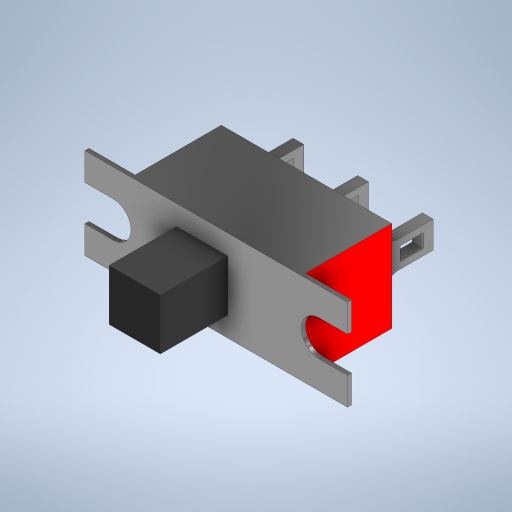
# Autodesk Inventor part: switch
Saved by Autodesk Inventor 2024 (Build 280153000, 153)
## iProperties
Created: 2023-11-08
Part Number: switch
Material: Všeobecné
Document SubType Name: Modeling
Designer: Simak
Density: 1 g/cm^3
Appearance: Výchozí
Author: Simak
Autodesk Inventor part; units mm, degrees
ref_plane "YZ Plane" through (0, 0, 0) normal (1, 0, 0) x (0, 1, 0)
ref_plane "XZ Plane" through (0, 0, 0) normal (0, 1, 0) x (-1, 0, 0)
ref_plane "XY Plane" through (0, 0, 0) normal (0, 0, 1) x (1, 0, 0)
sketch "Náčrt1" plane through (0, 0, 0) normal (0, 0, 1) x (1, 0, 0)
  line L0 (-6.325, 3.375) -> (6.325, 3.375)
  line L1 (6.325, 3.375) -> (6.325, -3.375)
  line L2 (6.325, -3.375) -> (-6.325, -3.375)
  line L3 (-6.325, -3.375) -> (-6.325, 3.375)
  line L4 (0, 0) -> (-6.325, 3.375) construction
  line L5 (6.325, 3.375) -> (0, 0) construction
  line L6 (6.325, -3.375) -> (0, 0) construction
  dimension "d0" = 12.65
  dimension "d1" = 6.75
  constraints: 14 end point, 2 equal length, 2 parallel, 1 horizontal, 1 perpendicular
  measures "d0" distance of L0.start L0.end
  measures "d1" distance of L0.end L1.end
extrude "Vysunutí1" add sketch "Náčrt1" along normal blind 6.4
sketch "Náčrt2" plane through (0, 0, 6.4) normal (0, 0, 1) x (1, 0, 0)
  line L0 (-9.75, 3.375) -> (9.75, 3.375)
  line L1 (9.75, 3.375) -> (9.75, -3.375)
  line L2 (9.75, -3.375) -> (-9.75, -3.375)
  line L3 (-9.75, -3.375) -> (-9.75, 3.375)
  line L4 (6.325, -3.375) -> (6.325, 3.375) projected
  line L5 (6.325, 0) -> (9.75, 0) construction
  line L6 (-9.75, 0) -> (-6.325, 0) construction
  line L7 (-6.325, 3.375) -> (-6.325, -3.375) projected
  point P0 (0, 0)
  dimension "d4" = 19.5
  constraints: 12 end point, 4 midpoint, 2 horizontal alignment, 2 parallel, 1 collinear, 1 horizontal, 1 perpendicular
  measures "d4" distance of L0.start L0.end
extrude "Vysunutí2" add sketch "Náčrt2" along normal blind 0.3
sketch "Náčrt3" plane through (0, 0, 6.7) normal (0, 0, 1) x (1, 0, 0)
  circle A0 centre (-7.65, 0) radius 1.325
  circle A1 centre (7.65, 0) radius 1.325
  line L0 (-6.325, 3.375) -> (-6.325, -3.375) projected
  line L1 (6.325, -3.375) -> (6.325, 3.375) projected
  line L2 (-7.65, 1.325) -> (-9.75, 1.325)
  line L3 (-9.75, 3.375) -> (-9.75, -3.375) projected
  line L4 (-7.65, -1.325) -> (-9.75, -1.325)
  line L5 (7.65, 1.325) -> (9.75, 1.325)
  line L6 (9.75, -3.375) -> (9.75, 3.375) projected
  line L7 (7.65, -1.325) -> (9.75, -1.325)
  point P0 (0, 0)
  dimension "d7" = 2.65
  constraints: 8 end point, 6 tangent, 4 point on circle, 4 point on line, 2 centre point, 2 horizontal, 2 horizontal alignment, 1 equal radius, 1 parallel, 1 perpendicular
  measures "d7" diameter of A0
extrude "Vysunutí3" cut sketch "Náčrt3" against normal up to surface (0.3 mm away)
sketch "Náčrt4" plane through (-6.325, -3.375, 0) normal (-1, 0, 0) x (0, 0, 1)
  line L0 (0, 0) -> (0, 6.75) projected
  line L1 (-1.5, 4.375) -> (-4.2, 4.375)
  line L2 (-4.2, 4.375) -> (-4.2, 2.375)
  line L3 (-4.2, 2.375) -> (-1.5, 2.375)
  line L4 (-3.45, 2.875) -> (-1.75, 2.875)
  line L5 (-1.75, 2.875) -> (-1.75, 3.875)
  line L6 (-1.75, 3.875) -> (-3.45, 3.875)
  line L7 (-3.45, 3.875) -> (-3.45, 2.875)
  line L8 (0, 0) -> (6.4, 0) projected
  line L9 (-4.2, 2.375) -> (0, 0) construction
  line L10 (-4.2, 4.375) -> (0, 6.75) construction
  line L11 (-1.5, 4.375) -> (-1, 4.525)
  line L12 (-1.5, 2.375) -> (-1, 2.225)
  line L13 (-1, 4.525) -> (-0.1, 4.525)
  line L14 (-0.1, 4.525) -> (-0.7641, 5.0796)
  arc A0 (-0.6648, 5.25) -> (-0.7641, 5.0796) centre (-0.7, 5.1564) ccw
  line L15 (-0.6648, 5.25) -> (0, 5)
  line L16 (-1, 2.225) -> (-0.1, 2.225)
  line L17 (-0.1, 2.225) -> (-0.7641, 1.6704)
  arc A1 (-0.7641, 1.6704) -> (-0.6648, 1.5) centre (-0.7, 1.5936) ccw
  line L18 (-0.6648, 1.5) -> (0, 1.75)
  line L19 (-0.1, 4.525) -> (0, 5) construction
  line L20 (-0.1, 2.225) -> (0, 1.75) construction
  point P0 (0, 3.375)
  dimension "d10" = 2
  dimension "d11" = 4.2
  dimension "d12" = 0.5
  dimension "d13" = 0.5
  dimension "d14" = 1.75
  dimension "d16" = 0.75
  dimension "d18" = 1.5
  dimension "d19" = 2.3
  dimension "d20" = 1
  dimension "d22" = 0.8
  dimension "d23" = 3.75
  dimension "d24" = 0.1
  dimension "d25" = 3.25
  dimension "d27" = 0.1
  constraints: 38 end point, 7 equal length, 4 point on circle, 4 tangent, 3 horizontal, 3 parallel, 3 perpendicular, 2 centre point, 2 point on line, 2 vertical alignment, 1 equal radius
  measures "d10" distance of L1.end L2.end
  measures "d11" distance between parallel lines of L0 L2
  measures "d12" distance between parallel lines of L1 L6
  measures "d13" distance between parallel lines of L3 L4
  measures "d14" distance between parallel lines of L0 L5
  measures "d16" distance between parallel lines of L2 L7
  measures "d18" distance from line of L0 L3.end
  measures "d19" distance of L12.end L11.end
  measures "d20" distance from line of L0 L11.end
  measures "d23" distance of L18.start L15.start
  measures "d24" distance from line of L0 L13.end
  measures "d25" distance of L15.end L18.end
  measures "d27" radius of A0
extrude "Vysunutí4" add sketch "Náčrt4" against normal up to surface (12.65 mm away)
sketch "Náčrt5" plane through (-6.325, -3.375, 0) normal (0, -1, 0) x (1, 0, 0)
  line L0 (12.65, 0) -> (12.65, 6.4) projected
  line L1 (12.65, 0) -> (11.525, 0)
  line L2 (11.525, 0) -> (11.525, -4.2)
  line L3 (11.525, -4.2) -> (12.65, -4.2)
  line L4 (12.65, -4.2) -> (12.65, 0)
  line L5 (0, 0) -> (12.65, 0) projected
  line L6 (10.725, -4.2) -> (6.725, -4.2)
  line L7 (6.725, -4.2) -> (6.725, 0)
  line L8 (6.725, 0) -> (10.725, 0)
  line L9 (10.725, 0) -> (10.725, -4.2)
  line L10 (5.925, -4.2) -> (1.925, -4.2)
  line L11 (1.925, -4.2) -> (1.925, 0)
  line L12 (1.925, 0) -> (5.925, 0)
  line L13 (5.925, 0) -> (5.925, -4.2)
  line L14 (1.125, -4.2) -> (0, -4.2)
  line L15 (0, -4.2) -> (0, 0)
  line L16 (0, 0) -> (1.125, 0)
  line L17 (1.125, 0) -> (1.125, -4.2)
  line L18 (0, -4.2) -> (12.65, -4.2) projected
  line L19 (11.525, -2.1) -> (10.725, -2.1) construction
  line L20 (6.725, -2.1) -> (5.925, -2.1) construction
  line L21 (1.925, -2.1) -> (1.125, -2.1) construction
  point P0 (6.325, 0)
  point P1 (1.125, 0)
  dimension "d30" = 0.8
  dimension "d31" = 4
  constraints: 38 end point, 8 parallel, 6 midpoint, 5 point on line, 4 collinear, 4 horizontal, 4 perpendicular
  measures "d30" distance of L20.start L20.end
  measures "d31" distance of L10.start L10.end
extrude "Vysunutí5" cut sketch "Náčrt5" against normal through all contours L4 L3 L2 L1 | L9 L6 L7 L5 | L13 L10 L11 L5 | L17 L14 L15 L5
sketch "Náčrt6" plane through (0, 0, 6.7) normal (0, 0, 1) x (1, 0, 0)
  line L0 (0.85, 1.9) -> (-2.95, 1.9)
  line L1 (-2.95, 1.9) -> (-2.95, -1.9)
  line L2 (-2.95, -1.9) -> (0.85, -1.9)
  line L3 (0.85, -1.9) -> (0.85, 1.9)
  line L4 (-9.75, -1.325) -> (-9.75, -3.375) projected
  point P0 (0, 0)
  point P1 (0.85, 0)
  dimension "d34" = 3.8
  dimension "d35" = 6.8
  constraints: 8 end point, 2 parallel, 2 perpendicular, 1 horizontal, 1 horizontal alignment, 1 midpoint
  measures "d34" distance of L1.end L2.end
  measures "d35" distance between parallel lines of L4 L1
extrude "Vysunutí6" add sketch "Náčrt6" along normal blind 5
